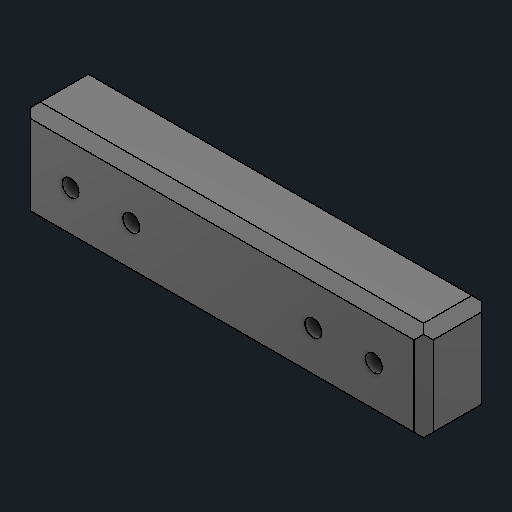
# Autodesk Inventor part: Extrusion Sides
Saved by Autodesk Inventor 2026.2 (Build 302298000, 298)
## iProperties
Created: 2026-07-24
Part Number: Extrusion Sides
Material: ABS Plastic
Document SubType Name: Modeling
Designer: JoshuaEah
Density: 1.06 g/cm^3
Appearance: Smooth - Black
Author: JoshuaEah
Autodesk Inventor part; units mm, degrees
ref_plane "YZ Plane" through (0, 0, 0) normal (1, 0, 0) x (0, 1, 0)
ref_plane "XZ Plane" through (0, 0, 0) normal (0, 1, 0) x (-1, 0, 0)
ref_plane "XY Plane" through (0, 0, 0) normal (0, 0, 1) x (1, 0, 0)
sketch "Sketch1" plane through (0, 0, 0) normal (0, 0, 1) x (1, 0, 0)
  line L0 (6.35, 6.35) -> (126.35, 6.35)
  line L1 (126.35, 6.35) -> (126.35, 26.35)
  line L2 (126.35, 26.35) -> (6.35, 26.35)
  line L3 (6.35, 26.35) -> (6.35, 6.35)
  line L4 (0, 0) -> (132.7, 0)
  line L5 (132.7, 0) -> (132.7, 32.7)
  line L6 (132.7, 32.7) -> (0, 32.7)
  line L7 (0, 32.7) -> (0, 0)
  line L8 (46.35, 26.35) -> (46.35, 6.35)
  line L9 (86.35, 26.35) -> (86.35, 6.35)
  line L10 (6.35, 16.35) -> (126.35, 16.35)
  point P0 (16.35, 16.35)
  point P1 (36.35, 16.35)
  point P2 (96.35, 16.35)
  point P3 (116.35, 16.35)
  dimension "d0" = 120
  dimension "d1" = 20
  dimension "d2" = 6.35
  dimension "d3" = 40
  dimension "d4" = 40
  dimension "d10" = 10
  dimension "d11" = 10
  dimension "d12" = 10
  dimension "d13" = 10
  constraints: 22 end point, 8 point on line, 4 parallel, 4 perpendicular, 2 midpoint, 1 coincident, 1 horizontal, 3 other
  measures "d0" distance of L1.end L2.end
  measures "d1" distance of L0.end L1.end
  measures "d2" distance between parallel lines of L3 L7
  measures "d3" distance between parallel lines of L3 L8
  measures "d4" distance between parallel lines of L1 L9
  measures "d10" distance from line of L3 point (16.35, 16.35)
  measures "d11" distance from line of L8 point (36.35, 16.35)
  measures "d12" distance from line of point (96.35, 16.35) L9
  measures "d13" distance from line of point (116.35, 16.35) L1
extrude "Extrusion1" add sketch "Sketch1" against normal blind 19.05 contours L3 L10 L8 L0 | L8 L10 L9 L0 | L3 L2 L8 L10 | L9 L10 L1 L0 | L8 L2 L9 L10 | L9 L2 L1 L10 | L7 L6 L5 L4
extrude "Extrusion3" add sketch "Sketch1" against normal blind 3.175 from surface at -19.05 contours L8 L10 L9 L0 | L8 L2 L9 L10 | L7 L6 L5 L4
chamfer "Chamfer1" distance 3.175 angle 45 12 edges at (66.35, 32.7, 0) (132.7, 32.7, -11.1125) (132.7, 16.35, 0) (132.7, 0, -11.1125) (66.35, 0, 0) (0, 16.35, 0) (0, 32.7, -11.1125) (0, 0, -11.1125) (66.35, 32.7, -22.225) (66.35, 0, -22.225) (0, 16.35, -22.225) (132.7, 16.35, -22.225)
hole "Hole1" at (16.35, 16.35, 0) at (36.35, 16.35, 0) at (96.35, 16.35, 0) at (116.35, 16.35, 0) direction (0, 0, -1) diameter 5.5118 end through all start extended yes clearance for "Socket Head Cap Screw" size "M5" standard "Ansi Metric M Profile"
thicken "Thicken1" operation cut thickness 0.1 both sides no extend neighbours yes toward (0, 1, 0) faces at (99.6833, 26.35, -20.1083) (86.35, 13.0167, -20.1083) (113.0167, 6.35, -20.1083) (126.35, 19.6833, -20.1083)
thicken "Thicken2" operation add thickness 0.1 both sides no extend neighbours yes toward (1, 0, 0) faces at (46.35, 19.6833, -20.1083) (19.6833, 26.35, -20.1083) (6.35, 13.0167, -20.1083) (33.0167, 6.35, -20.1083)
equation "\"d4\" = d3"
equation "\"d11\" = d10"
equation "\"d12\" = d10"
equation "\"d13\" = d10"
body "Solid1"
